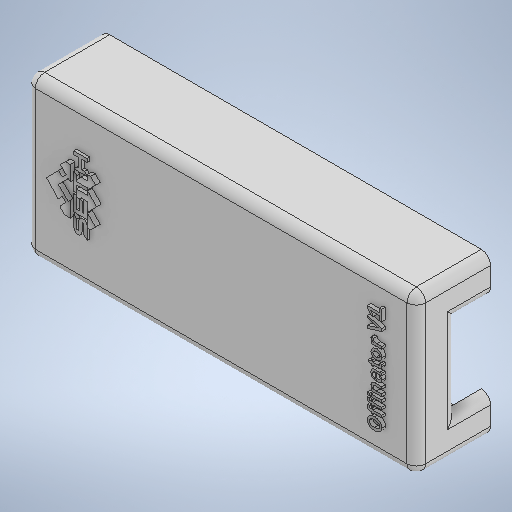
# Autodesk Inventor part: top part
Saved by Autodesk Inventor 2025.2 (Build 292293000, 293)
## iProperties
Created: 2026-01-28
Part Number: top part
Material: Generic
Document SubType Name: Modeling
Designer: seths
Density: 1 g/cm^3
Appearance: Default
Author: seths
Autodesk Inventor part; units mm, degrees
ref_plane "YZ Plane" through (0, 0, 0) normal (1, 0, 0) x (0, 1, 0)
ref_plane "XZ Plane" through (0, 0, 0) normal (0, 1, 0) x (-1, 0, 0)
ref_plane "XY Plane" through (0, 0, 0) normal (0, 0, 1) x (1, 0, 0)
sketch "Sketch1" plane through (0, 0, 0) normal (0, 0, 1) x (1, 0, 0)
  line L0 (-40, 15) -> (0, 15)
  line L1 (0, 15) -> (0, 0)
  line L2 (-41, 16) -> (1, 16)
  line L3 (1, 16) -> (1, -1)
  line L4 (-34.585, 0) -> (-34.585, -1)
  line L5 (-31, 0) -> (-31, -1)
  line L6 (0, 0) -> (-31, 0)
  line L7 (-34.585, 0) -> (-40, 0)
  line L8 (1, -1) -> (-31, -1)
  line L9 (-34.585, -1) -> (-41, -1)
  line L10 (0, 12) -> (1, 12)
  line L11 (0, 3) -> (1, 3)
  line L12 (-41, 9.5362) -> (-40, 9.5362)
  line L13 (-41, 6.9849) -> (-40, 6.9849)
  line L14 (-40, 0) -> (-40, 6.9849)
  line L15 (-40, 9.5362) -> (-40, 15)
  line L16 (-41, -1) -> (-41, 6.9849)
  line L17 (-41, 9.5362) -> (-41, 16)
  point P0 (-15, -1)
  point P1 (-15.5, 0)
  dimension "d0" = 40
  dimension "d1" = 42
  dimension "d4" = 1
  dimension "d6" = 5.415
  dimension "d8" = 4
  dimension "d9" = 4
  dimension "d21" = 17
  dimension "d22" = 17
  dimension "d25" = 15
  dimension "d26" = 1
  dimension "d27" = 32
  constraints: 36 end point, 18 perpendicular, 8 parallel, 4 horizontal, 4 point on line, 2 midpoint
  measures "d0" distance of L0.start L0.end
  measures "d1" distance of L2.start L2.end
  measures "d4" distance between parallel lines of L2 L0
  measures "d6" distance from line of L4 L7.end
  measures "d8" distance from line of L10 L2.end
  measures "d9" distance from line of L11 L3.end
  measures "d21" distance of L2.end L3.end
  measures "d22" distance of L2.start L9.end
  measures "d25" distance of L0.end L1.end
  measures "d26" distance between parallel lines of L6 L8
  measures "d27" distance of L3.end L5.end
extrude "Extrusion1" add sketch "Sketch1" along normal blind 7 contours L15 L12 L17 L2 L3 L10 L1 L0 | L11 L3 L8 L5 L6 L1 | L4 L9 L16 L13 L14 L7
sketch "Sketch2" plane through (-31, -1, 0) normal (-1, 0, 0) x (0, 0, 1)
  line L0 (0, 0) -> (7, 0) projected
  line L1 (7, 1) -> (3.5058, 1)
  line L2 (3.5058, 1) -> (3.5058, 0)
  line L3 (3.5058, 0) -> (7, 0)
  line L4 (7, 0) -> (7, 1)
  point P0 (0, 1)
  constraints: 8 end point, 2 parallel, 1 horizontal, 1 perpendicular, 1 point on line
extrude "Extrusion2" add sketch "Sketch2" along normal blind 8
sketch "Sketch3" plane through (0, 12, 0) normal (0, -1, 0) x (1, 0, 0)
  line L0 (0, 0) -> (0, 7) projected
  line L1 (1, 0) -> (1, 7) projected
  line L2 (0, 7) -> (1, 7)
  line L3 (1, 7) -> (1, 3.627)
  line L4 (1, 3.627) -> (0, 3.627)
  line L5 (0, 3.627) -> (0, 7)
  point P0 (0, 3.627)
  constraints: 8 end point, 2 parallel, 1 horizontal, 1 perpendicular, 1 point on line
extrude "Extrusion3" add sketch "Sketch3" along normal blind 12
sketch "Sketch4" plane through (-41, 9.5362, 0) normal (0, -1, 0) x (1, 0, 0)
  line L0 (1, 0) -> (1, 7) projected
  line L1 (0, 0) -> (1, 0)
  line L2 (1, 0) -> (1, 2.6982)
  line L3 (1, 2.6982) -> (0, 2.6982)
  line L4 (0, 2.6982) -> (0, 0)
  line L5 (0, 7) -> (1, 7)
  line L6 (1, 7) -> (1, 5.3298)
  line L7 (1, 5.3298) -> (0, 5.3298)
  line L8 (0, 5.3298) -> (0, 7)
  point P0 (41, 0)
  constraints: 16 end point, 4 parallel, 3 point on line, 2 horizontal, 2 perpendicular
extrude "Extrusion4" add sketch "Sketch4" along normal blind 10
sketch "Sketch5" plane through (0, 0, 7) normal (0, 0, 1) x (1, 0, 0)
  line L0 (-41, -1) -> (1, -1) projected
  line L1 (-41, 16) -> (-41, -1) projected
  line L2 (1, -1) -> (-41, -1)
  line L3 (-41, -1) -> (-41, 16)
  line L4 (-41, 16) -> (1, 16)
  line L5 (1, 16) -> (1, -1)
  point P0 (0, 0)
  point P1 (-40, -1)
  point P2 (0, -1)
  point P3 (-41, -1)
  point P4 (0, -1)
  constraints: 8 end point, 2 parallel, 1 horizontal, 1 perpendicular
extrude "Extrusion5" add sketch "Sketch5" along normal blind 1
fillet "Fillet1" radius 1 18 edges at (-41, 7.5, 8) (-20, -1, 8) (-41, -1, 4) (1, -1, 4) (1, 7.5, 8) (-20, 16, 8) (-41, 16, 4) (-41, 8.2605, 5.3298) (-41, 6.9849, 4.014) (-41, 8.2605, 2.6982) (-41, 9.5362, 4.014) (1, 16, 4) (-32.7925, -1, 3.5058) (-31, -1, 1.7529) (-34.585, -1, 1.7529) (1, 7.5, 3.627) (1, 12, 1.8135) (1, 3, 1.8135)
sketch "Sketch6" plane through (0, 0, 8) normal (0, 0, 1) x (1, 0, 0)
  line L0 (-35.5627, 5.6762) -> (-35.2348, 5.3432)
  line L1 (-35.2348, 5.3432) -> (-35.2348, 4.4056)
  line L2 (-35.5627, 5.6762) -> (-35.5627, 4.3672)
  line L3 (-35.0235, 4.4056) -> (-35.0235, 5.3227)
  line L4 (-34.4741, 4.2673) -> (-34.4741, 5.2868)
  line L5 (-34.4741, 5.2868) -> (-34.6739, 5.2868)
  line L6 (-34.6739, 5.2868) -> (-34.6739, 4.3672)
  line L7 (-34.6739, 4.3672) -> (-34.6739, 5.2868)
  line L8 (-34.4741, 4.2673) -> (-34.1245, 3.9123)
  line L9 (-34.1245, 3.9123) -> (-34.1245, 5.3227)
  arc A0 (-35.5627, 4.4056) -> (-34.6739, 4.4056) centre (-35.1183, 4.4056) ccw
  line L10 (-35.2348, 4.4056) -> (-35.2348, 4.3672)
  line L11 (-35.0235, 4.4056) -> (-35.0235, 4.3672)
  line L12 (-34.6756, 4.3672) -> (-34.6739, 4.3672)
  line L13 (-35.5627, 4.3672) -> (-35.561, 4.3672)
  line L14 (-35.2348, 4.3672) -> (-35.0235, 4.3672)
  arc A1 (-34.1245, 5.2868) -> (-35.0235, 5.2868) centre (-34.574, 5.2868) ccw
  line L15 (-35.5627, 7.5605) -> (-35.5627, 5.8491)
  line L16 (-35.5627, 5.8491) -> (-34.1245, 5.8491)
  line L17 (-34.1245, 5.8491) -> (-34.1245, 7.5605)
  line L18 (-34.1245, 7.5605) -> (-34.4741, 7.5605)
  line L19 (-34.4741, 7.5605) -> (-34.4741, 6.4201)
  line L20 (-34.6739, 6.4201) -> (-34.6756, 6.4201)
  line L21 (-34.6756, 6.4201) -> (-34.6756, 7.2854)
  line L22 (-34.6756, 7.2854) -> (-34.8436, 7.4444)
  line L23 (-34.8436, 7.4444) -> (-34.994, 7.2854)
  line L24 (-34.994, 7.2854) -> (-34.994, 6.2361)
  line L25 (-34.994, 6.2361) -> (-35.2348, 6.2361)
  line L26 (-35.2348, 6.2361) -> (-35.2348, 7.5605)
  line L27 (-35.2348, 7.5605) -> (-35.5627, 7.5605)
  line L28 (-34.4741, 6.4201) -> (-34.4741, 6.2361)
  line L29 (-34.6756, 6.4201) -> (-34.6756, 6.2361)
  line L30 (-34.6756, 6.2361) -> (-34.4741, 6.2361)
  line L31 (-35.5627, 7.7606) -> (-35.5627, 9.686)
  line L32 (-35.5627, 9.686) -> (-35.2348, 9.4068)
  line L33 (-35.2348, 9.4068) -> (-35.2348, 8.8484)
  line L34 (-35.2348, 8.8484) -> (-34.1245, 8.8484)
  line L35 (-34.1245, 8.8484) -> (-34.1245, 8.5112)
  line L36 (-34.1245, 8.5112) -> (-35.2348, 8.5112)
  line L37 (-35.2348, 8.5112) -> (-35.2348, 7.7606)
  line L38 (-35.2348, 7.7606) -> (-35.5627, 7.7606)
  line L39 (-35.0438, 7.5876) -> (-35.0438, 8.348)
  line L40 (-35.0438, 8.348) -> (-33.9052, 8.348)
  line L41 (-33.9052, 8.348) -> (-33.9052, 9.0188)
  line L42 (-33.9052, 9.0188) -> (-35.0235, 9.0188)
  line L43 (-35.0235, 9.0188) -> (-35.0235, 9.2268)
  line L44 (-35.0235, 9.2268) -> (-34.5748, 9.686)
  line L45 (-34.5748, 9.686) -> (-33.9052, 9.686)
  line L46 (-33.9052, 9.686) -> (-33.9052, 10.2697)
  line L47 (-33.9052, 10.2697) -> (-33.5565, 10.2697)
  line L48 (-33.5565, 10.2697) -> (-33.0182, 9.723)
  line L49 (-33.0182, 9.723) -> (-33.8726, 8.8484)
  line L50 (-33.8726, 8.8484) -> (-33.8726, 8.7417)
  line L51 (-33.8726, 8.7417) -> (-32.9067, 7.7606)
  line L52 (-32.9067, 7.7606) -> (-33.8726, 6.7719)
  line L53 (-33.8726, 6.7719) -> (-33.8726, 6.6844)
  line L54 (-33.8726, 6.6844) -> (-33.0182, 5.8166)
  line L55 (-33.0182, 5.8166) -> (-33.5565, 5.2865)
  line L56 (-33.5565, 5.2865) -> (-33.9052, 5.2865)
  line L57 (-33.9052, 5.2865) -> (-33.9052, 7.7435)
  line L58 (-33.9052, 7.7435) -> (-34.5445, 7.7606)
  line L59 (-34.5445, 7.7606) -> (-34.6919, 7.5876)
  line L60 (-34.6919, 7.5876) -> (-35.0438, 7.5876)
  line L61 (-35.5627, 9.8728) -> (-34.0987, 9.8728)
  line L62 (-34.0987, 9.8728) -> (-34.4034, 10.2217)
  line L63 (-34.4034, 10.2217) -> (-34.6919, 10.2217)
  line L64 (-34.6919, 10.2217) -> (-34.6919, 11.177)
  line L65 (-34.6919, 11.177) -> (-34.1331, 11.177)
  line L66 (-34.1331, 11.177) -> (-34.1331, 11.5423)
  line L67 (-34.1331, 11.5423) -> (-35.5568, 11.5423)
  line L68 (-35.5568, 11.5423) -> (-35.5568, 11.177)
  line L69 (-35.5568, 11.177) -> (-35.0438, 11.177)
  line L70 (-35.0438, 11.177) -> (-35.0235, 10.2217)
  line L71 (-35.0235, 10.2217) -> (-35.2348, 10.2217)
  line L72 (-35.2348, 10.2217) -> (-35.5627, 9.8728)
  line L73 (-35.746, 5.2733) -> (-36.3259, 5.2865)
  line L74 (-36.3259, 5.2865) -> (-36.8281, 5.7616)
  line L75 (-36.8281, 5.7616) -> (-36.825, 5.8944)
  line L76 (-36.825, 5.8944) -> (-35.746, 6.9444)
  line L77 (-35.746, 8.6664) -> (-36.7984, 9.7479)
  line L78 (-36.7984, 9.7479) -> (-36.2603, 10.2777)
  line L79 (-36.2603, 10.2777) -> (-35.746, 10.2887)
  line L80 (-35.746, 6.9444) -> (-35.746, 10.2887)
  line L81 (-35.9563, 6.7398) -> (-37.0278, 7.7788)
  line L82 (-37.0278, 7.7788) -> (-35.9569, 8.8831)
  line L83 (-36.1731, 9.1054) -> (-36.5951, 8.6948)
  line L84 (-36.5951, 8.6948) -> (-36.9994, 9.1102)
  line L85 (-36.9994, 9.1102) -> (-38.2936, 7.7756)
  line L86 (-38.2936, 7.7756) -> (-37.046, 6.4271)
  line L87 (-37.046, 6.4271) -> (-36.6057, 6.8875)
  line L88 (-36.6057, 6.8875) -> (-36.2161, 6.487)
  line L89 (-35.746, 6.9444) -> (-35.746, 5.2733)
  point P0 (0, 0)
  point P1 (-10.6987, 14.8672)
  point P2 (-34.6739, 4.4056)
  constraints: 180 end point, 45 perpendicular, 29 point on line, 13 parallel, 6 point on circle, 4 tangent, 2 centre point, 1 collinear, 1 midpoint
extrude "Extrusion6" add sketch "Sketch6" along normal blind 0.5 contours L39 L40 L41 L42 L43 L44 L45 L46 L47 L48 L49 L50 L51 L52 L53 L54 L55 L56 L57 L58 L59 L60 | L73 L74 L75 L76 L89 | L76 L88 L87 L86 L85 L84 L83 L77 L82 L81 | L77 L78 L79 L80
extrude "Extrusion7" add sketch "Sketch6" along normal blind 0.3 contours L0 L1 L10 L14 L11 L3 A1 L9 L8 L4 L5 L6 A0 L2 | L27 L26 L25 L24 L23 L22 L21 L29 L30 L28 L19 L18 L17 L16 L15 | L31 L32 L33 L34 L35 L36 L37 L38 | L72 L71 L70 L69 L68 L67 L66 L65 L64 L63 L62 L61
sketch "Sketch7" plane through (0, 0, 8) normal (0, 0, 1) x (1, 0, 0)
  spline S0 degree 2 poles (-2.3046, 2.3895) (-2.3046, 2.0856) (-2.7606, 1.7474) (-3.0963, 1.7474) knots 0 0 0 1 2 2 2
  spline S1 degree 2 poles (-3.0963, 1.7474) (-3.4294, 1.7474) (-3.8765, 2.1071) (-3.8765, 2.4022) knots 0 0 0 1 2 2 2
  spline S2 degree 2 poles (-3.8765, 2.4022) (-3.8765, 2.6986) (-3.4294, 3.0444) (-3.0925, 3.0444) knots 0 0 0 1 2 2 2
  spline S3 degree 2 poles (-3.0925, 3.0444) (-2.7404, 3.0444) (-2.3046, 2.6859) (-2.3046, 2.3895) knots 0 0 0 1 2 2 2
  spline S4 degree 2 poles (-2.5263, 2.3921) (-2.5263, 2.5403) (-2.772, 2.7455) (-3.095, 2.7455) knots 0 0 0 1 2 2 2
  spline S5 degree 2 poles (-3.095, 2.7455) (-3.3572, 2.7455) (-3.6561, 2.5757) (-3.6561, 2.3971) knots 0 0 0 1 2 2 2
  spline S6 degree 2 poles (-3.6561, 2.3971) (-3.6561, 2.0438) (-3.0874, 2.0438) knots 0 0 0 1 1 1
  spline S7 degree 2 poles (-3.0874, 2.0438) (-2.8113, 2.0438) (-2.5263, 2.2236) (-2.5263, 2.3921) knots 0 0 0 1 2 2 2
  line L0 (-2.3287, 3.57) -> (-2.3287, 3.3243)
  line L1 (-2.3287, 3.3243) -> (-3.2597, 3.3243)
  line L2 (-3.2597, 3.3243) -> (-3.2597, 3.1558)
  line L3 (-3.2597, 3.1558) -> (-3.4573, 3.1558)
  line L4 (-3.4573, 3.1558) -> (-3.4573, 3.3243)
  line L5 (-3.4573, 3.3243) -> (-3.513, 3.3243)
  spline S8 degree 2 poles (-3.513, 3.3243) (-3.6776, 3.3243) (-3.879, 3.4852) (-3.879, 3.7296) knots 0 0 0 1 2 2 2
  spline S9 degree 2 poles (-3.879, 3.7296) (-3.879, 3.7651) (-3.8765, 3.8196) knots 0 0 0 1 1 1
  line L6 (-3.8765, 3.8196) -> (-3.6764, 3.8196)
  spline S10 degree 2 poles (-3.6764, 3.8196) (-3.6802, 3.7714) (-3.6802, 3.7537) knots 0 0 0 1 1 1
  spline S11 degree 2 poles (-3.6802, 3.7537) (-3.6802, 3.66) (-3.6295, 3.584) (-3.5624, 3.57) (-3.4573, 3.57) knots 0 0 0 1 2 3 3 3
  line L7 (-3.4573, 3.57) -> (-3.4573, 3.8196)
  line L8 (-3.4573, 3.8196) -> (-3.2597, 3.8196)
  line L9 (-3.2597, 3.8196) -> (-3.2597, 3.57)
  line L10 (-3.2597, 3.57) -> (-2.3287, 3.57)
  line L11 (-2.3287, 4.2933) -> (-2.3287, 4.0475)
  line L12 (-2.3287, 4.0475) -> (-3.2597, 4.0475)
  line L13 (-3.2597, 4.0475) -> (-3.2597, 3.8791)
  line L14 (-3.2597, 3.8791) -> (-3.4573, 3.8791)
  line L15 (-3.4573, 3.8791) -> (-3.4573, 4.0475)
  line L16 (-3.4573, 4.0475) -> (-3.513, 4.0475)
  spline S12 degree 2 poles (-3.513, 4.0475) (-3.6776, 4.0475) (-3.879, 4.2084) (-3.879, 4.4529) knots 0 0 0 1 2 2 2
  spline S13 degree 2 poles (-3.879, 4.4529) (-3.879, 4.4883) (-3.8765, 4.5428) knots 0 0 0 1 1 1
  line L17 (-3.8765, 4.5428) -> (-3.6764, 4.5428)
  spline S14 degree 2 poles (-3.6764, 4.5428) (-3.6802, 4.4947) (-3.6802, 4.4769) knots 0 0 0 1 1 1
  spline S15 degree 2 poles (-3.6802, 4.4769) (-3.6802, 4.3832) (-3.6295, 4.3072) (-3.5624, 4.2933) (-3.4573, 4.2933) knots 0 0 0 1 2 3 3 3
  line L18 (-3.4573, 4.2933) -> (-3.4573, 4.5428)
  line L19 (-3.4573, 4.5428) -> (-3.2597, 4.5428)
  line L20 (-3.2597, 4.5428) -> (-3.2597, 4.2933)
  line L21 (-3.2597, 4.2933) -> (-2.3287, 4.2933)
  line L22 (-2.3287, 4.9848) -> (-2.3287, 4.7302)
  line L23 (-2.3287, 4.7302) -> (-3.4573, 4.7302)
  line L24 (-3.4573, 4.7302) -> (-3.4573, 4.9848)
  line L25 (-3.4573, 4.9848) -> (-2.3287, 4.9848)
  line L26 (-3.589, 4.9848) -> (-3.589, 4.7302)
  line L27 (-3.589, 4.7302) -> (-3.8537, 4.7302)
  line L28 (-3.8537, 4.7302) -> (-3.8537, 4.9848)
  line L29 (-3.8537, 4.9848) -> (-3.589, 4.9848)
  line L30 (-2.3287, 6.2248) -> (-2.3287, 5.9703)
  line L31 (-2.3287, 5.9703) -> (-3.0329, 5.9703)
  spline S16 degree 2 poles (-3.0329, 5.9703) (-3.1457, 5.9703) (-3.2584, 5.8677) (-3.2584, 5.7955) knots 0 0 0 1 2 2 2
  spline S17 degree 2 poles (-3.2584, 5.7955) (-3.2584, 5.6954) (-3.0836, 5.5459) (-2.9088, 5.5459) knots 0 0 0 1 2 2 2
  line L32 (-2.9088, 5.5459) -> (-2.3287, 5.5459)
  line L33 (-2.3287, 5.5459) -> (-2.3287, 5.2914)
  line L34 (-2.3287, 5.2914) -> (-3.4573, 5.2914)
  line L35 (-3.4573, 5.2914) -> (-3.4573, 5.5231)
  line L36 (-3.4573, 5.5231) -> (-3.1951, 5.5231)
  spline S18 degree 2 poles (-3.1951, 5.5231) (-3.4801, 5.6447) (-3.4801, 5.8651) knots 0 0 0 1 1 1
  spline S19 degree 2 poles (-3.4801, 5.8651) (-3.4801, 6.0133) (-3.2926, 6.2248) (-3.057, 6.2248) knots 0 0 0 1 2 2 2
  line L37 (-3.057, 6.2248) -> (-2.3287, 6.2248)
  line L38 (-2.3287, 7.4953) -> (-2.3287, 7.2521)
  spline S20 degree 2 poles (-2.3287, 7.2521) (-2.4313, 7.2204) (-2.5567, 7.2141) knots 0 0 0 1 1 1
  spline S21 degree 2 poles (-2.5567, 7.2141) (-2.3046, 7.1115) (-2.3046, 6.8316) knots 0 0 0 1 1 1
  spline S22 degree 2 poles (-2.3046, 6.8316) (-2.3046, 6.6631) (-2.5035, 6.4579) (-2.653, 6.4579) knots 0 0 0 1 2 2 2
  spline S23 degree 2 poles (-2.653, 6.4579) (-3.0418, 6.4579) (-3.0418, 7.1406) knots 0 0 0 1 1 1
  spline S24 degree 2 poles (-3.0418, 7.1406) (-3.0418, 7.1672) (-3.0405, 7.2141) knots 0 0 0 1 1 1
  line L39 (-3.0405, 7.2141) -> (-3.1254, 7.2141)
  spline S25 degree 2 poles (-3.1254, 7.2141) (-3.3002, 7.2141) (-3.3002, 6.9747) knots 0 0 0 1 1 1
  spline S26 degree 2 poles (-3.3002, 6.9747) (-3.3002, 6.7416) (-3.1254, 6.7112) knots 0 0 0 1 1 1
  line L40 (-3.1254, 6.7112) -> (-3.1571, 6.4946)
  spline S27 degree 2 poles (-3.1571, 6.4946) (-3.2977, 6.5124) (-3.4801, 6.767) (-3.4801, 7.0076) knots 0 0 0 1 2 2 2
  spline S28 degree 2 poles (-3.4801, 7.0076) (-3.4801, 7.1381) (-3.437, 7.304) (-3.3331, 7.418) (-3.2115, 7.4611) (-3.0659, 7.4611) knots 0 0 0 1 2 3 4 4 4
  line L41 (-3.0659, 7.4611) -> (-2.5567, 7.4611)
  spline S29 degree 2 poles (-2.5567, 7.4611) (-2.4465, 7.4611) (-2.3287, 7.4953) knots 0 0 0 1 1 1
  spline S30 degree 2 poles (-2.9025, 7.2141) (-2.9025, 6.7201) (-2.6669, 6.7201) knots 0 0 0 1 1 1
  spline S31 degree 2 poles (-2.6669, 6.7201) (-2.5972, 6.7201) (-2.4972, 6.8189) (-2.4972, 6.9202) knots 0 0 0 1 2 2 2
  spline S32 degree 2 poles (-2.4972, 6.9202) (-2.4972, 7.0646) (-2.6821, 7.2141) (-2.7986, 7.2141) knots 0 0 0 1 2 2 2
  line L42 (-2.7986, 7.2141) -> (-2.9025, 7.2141)
  line L43 (-2.5276, 8.2894) -> (-2.3287, 8.2894)
  spline S33 degree 2 poles (-2.3287, 8.2894) (-2.3046, 8.1754) (-2.3046, 8.1121) knots 0 0 0 1 1 1
  spline S34 degree 2 poles (-2.3046, 8.1121) (-2.3046, 8.0095) (-2.3857, 7.8626) (-2.5276, 7.7942) (-2.6745, 7.7942) knots 0 0 0 1 2 3 3 3
  line L44 (-2.6745, 7.7942) -> (-3.2597, 7.7942)
  line L45 (-3.2597, 7.7942) -> (-3.2597, 7.6536)
  line L46 (-3.2597, 7.6536) -> (-3.4573, 7.6536)
  line L47 (-3.4573, 7.6536) -> (-3.4573, 7.8081)
  line L48 (-3.4573, 7.8081) -> (-3.7511, 7.8322)
  line L49 (-3.7511, 7.8322) -> (-3.7701, 8.0412)
  line L50 (-3.7701, 8.0412) -> (-3.4573, 8.0412)
  line L51 (-3.4573, 8.0412) -> (-3.4573, 8.2679)
  line L52 (-3.4573, 8.2679) -> (-3.2597, 8.2679)
  line L53 (-3.2597, 8.2679) -> (-3.2597, 8.0412)
  line L54 (-3.2597, 8.0412) -> (-2.7087, 8.0412)
  spline S35 degree 2 poles (-2.7087, 8.0412) (-2.6023, 8.0412) (-2.525, 8.1184) (-2.525, 8.2248) knots 0 0 0 1 2 2 2
  spline S36 degree 2 poles (-2.525, 8.2248) (-2.525, 8.2552) (-2.5276, 8.2894) knots 0 0 0 1 1 1
  spline S37 degree 2 poles (-2.3046, 8.9443) (-2.3046, 8.6947) (-2.6644, 8.4313) (-2.8974, 8.4313) knots 0 0 0 1 2 2 2
  spline S38 degree 2 poles (-2.8974, 8.4313) (-3.1469, 8.4313) (-3.4801, 8.7226) (-3.4801, 8.9607) knots 0 0 0 1 2 2 2
  spline S39 degree 2 poles (-3.4801, 8.9607) (-3.4801, 9.1874) (-3.1558, 9.48) (-2.8974, 9.48) knots 0 0 0 1 2 2 2
  spline S40 degree 2 poles (-2.8974, 9.48) (-2.6302, 9.48) (-2.3046, 9.1773) (-2.3046, 8.9443) knots 0 0 0 1 2 2 2
  spline S41 degree 2 poles (-2.5149, 8.9531) (-2.5149, 9.2102) (-2.8987, 9.2102) knots 0 0 0 1 1 1
  spline S42 degree 2 poles (-2.8987, 9.2102) (-3.0709, 9.2102) (-3.2711, 9.0874) (-3.2711, 8.9595) knots 0 0 0 1 2 2 2
  spline S43 degree 2 poles (-3.2711, 8.9595) (-3.2711, 8.8277) (-3.0646, 8.7011) (-2.8936, 8.7011) knots 0 0 0 1 2 2 2
  spline S44 degree 2 poles (-2.8936, 8.7011) (-2.71, 8.7011) (-2.5149, 8.8366) (-2.5149, 8.9531) knots 0 0 0 1 2 2 2
  line L55 (-2.3287, 9.9677) -> (-2.3287, 9.7131)
  line L56 (-2.3287, 9.7131) -> (-3.4573, 9.7131)
  line L57 (-3.4573, 9.7131) -> (-3.4573, 9.9423)
  line L58 (-3.4573, 9.9423) -> (-3.1875, 9.9423)
  spline S45 degree 2 poles (-3.1875, 9.9423) (-3.3445, 9.9917) (-3.4902, 10.164) (-3.4902, 10.2552) knots 0 0 0 1 2 2 2
  spline S46 degree 2 poles (-3.4902, 10.2552) (-3.4902, 10.2666) (-3.4889, 10.2881) knots 0 0 0 1 1 1
  line L59 (-3.4889, 10.2881) -> (-3.2153, 10.2881)
  spline S47 degree 2 poles (-3.2153, 10.2881) (-3.2153, 10.0943) (-2.9671, 9.9677) (-2.8518, 9.9677) knots 0 0 0 1 2 2 2
  line L60 (-2.8518, 9.9677) -> (-2.3287, 9.9677)
  line L61 (-2.3287, 11.6447) -> (-2.3287, 11.366)
  line L62 (-2.3287, 11.366) -> (-3.8537, 10.8961)
  line L63 (-3.8537, 10.8961) -> (-3.8537, 11.1862)
  line L64 (-3.8537, 11.1862) -> (-2.6846, 11.5357)
  line L65 (-2.6846, 11.5357) -> (-3.8537, 11.8929)
  line L66 (-3.8537, 11.8929) -> (-3.8537, 12.1222)
  line L67 (-3.8537, 12.1222) -> (-2.3287, 11.6447)
  line L68 (-2.3287, 13.4509) -> (-2.3287, 12.283)
  line L69 (-2.3287, 12.283) -> (-2.5529, 12.283)
  line L70 (-2.5529, 12.283) -> (-2.5529, 12.7428)
  line L71 (-2.5529, 12.7428) -> (-3.5155, 12.7428)
  spline S48 degree 2 poles (-3.5155, 12.7428) (-3.3167, 12.5136) (-3.2407, 12.3261) knots 0 0 0 1 1 1
  line L72 (-3.2407, 12.3261) -> (-3.5155, 12.3261)
  spline S49 degree 2 poles (-3.5155, 12.3261) (-3.589, 12.5174) (-3.6498, 12.6136) (-3.817, 12.7986) (-3.8841, 12.8366) knots 0 0 0 1 2 3 3 3
  line L73 (-3.8841, 12.8366) -> (-3.8841, 13.0202)
  line L74 (-3.8841, 13.0202) -> (-2.5529, 13.0202)
  line L75 (-2.5529, 13.0202) -> (-2.5529, 13.4509)
  line L76 (-2.5529, 13.4509) -> (-2.3287, 13.4509)
  point P0 (0, 0)
  point P1 (-3.8841, 1.66)
  constraints: 1 other
extrude "Extrusion8" add sketch "Sketch7" along normal blind 0.4
body "Solid1"
